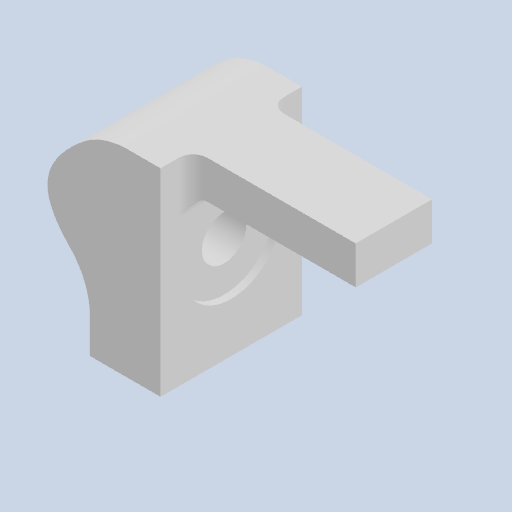
# Autodesk Inventor part: upor
Saved by Autodesk Inventor 2022 (Build 260153000, 153)
## iProperties
Created: 2024-12-11
Part Number: upor
Material: Типовые
Document SubType Name: Modeling
Designer: Andrey
Density: 1 g/cm^3
Appearance: По умолчанию
Author: Andrey
Autodesk Inventor part; units mm, degrees
ref_plane "YZ Plane" through (0, 0, 0) normal (1, 0, 0) x (0, 1, 0)
ref_plane "XZ Plane" through (0, 0, 0) normal (0, 1, 0) x (-1, 0, 0)
ref_plane "XY Plane" through (0, 0, 0) normal (0, 0, 1) x (1, 0, 0)
sketch "Эскиз1" plane through (0, 0, 0) normal (0, 0, 1) x (1, 0, 0)
  spline S0 degree 2 poles (0, -10.75) (-6, -5.75) (0, -0.75) knots -1 -1 -1 0 0 0
  circle A0 centre (31, -8.75) radius 2.1
  circle A1 centre (0.3533, 10.75) radius 2.1
  circle A2 centre (-6.5719, -8.75) radius 2.1
  arc A3 (26, -0.75) -> (0.0249, 0.0543) centre (13, -0.75) ccw
  line L0 (26, -0.75) -> (26, -14.75)
  line L1 (26, -14.75) -> (42.8533, -14.75)
  line L2 (42.8533, -14.75) -> (25.4056, 8.5426)
  arc A4 (25.4056, 8.5426) -> (13, 14.75) centre (13, -0.75) ccw
  line L3 (13, 14.75) -> (-7.8522, 14.75)
  line L4 (-7.8522, 14.75) -> (-8.8, 13.8022)
  arc A5 (-8.8, 13.8022) -> (-9.3554, 12.7353) centre (-7.3858, 12.388) ccw
  line L5 (-9.3554, 12.7353) -> (-9.4563, 12.1627)
  line L6 (-9.4563, 12.1627) -> (-3.6467, 12.1627)
  line L7 (-3.6467, 12.1627) -> (-3.6467, 9.9627)
  line L8 (-3.6467, 9.9627) -> (-9.8443, 9.9627)
  line L9 (-9.8443, 9.9627) -> (-13.8491, -12.75)
  line L10 (-13.8491, -12.75) -> (-7.0093, -12.75)
  line L11 (-7.0093, -12.75) -> (-7.0093, -14.75)
  line L12 (-7.0093, -14.75) -> (0, -14.75)
  line L13 (0, -14.75) -> (0, -11.6512)
  line L14 (1.5, -14.75) -> (26, -14.75)
  line L15 (0.9603, -9.5977) -> (1.5, -10.0794)
  line L16 (1.5, -10.0794) -> (1.5, -14.75)
  line L17 (0.9603, -1.9023) -> (2.3298, -0.75)
  line L18 (2.3298, -0.75) -> (26, -0.75)
  spline S1 degree 3 poles (0.0249, 0.0543) (0.0092, -0.1986) (-0.0544, -0.4464) (-0.2708, -0.9048) (-0.4215, -1.1114) (-0.6069, -1.2843) knots 0 0 0 0 0.5 0.5 1 1 1 1
  spline S2 degree 3 poles (-0.6318, -10.1924) (-0.4418, -10.3706) (-0.2885, -10.5841) (-0.1211, -10.951) (-0.0759, -11.0869) (-0.0153, -11.366) (0, -11.5084) (0, -11.6512) knots 0 0 0 0 0.476947 0.476947 0.738474 0.738474 1 1 1 1
  spline S3 degree 2 poles (-0.6318, -10.1924) (-5.3806, -5.7383) (-0.6069, -1.2843) knots -0.944242 -0.944242 -0.944242 -0.053426 -0.053426 -0.053426
  line L19 (1.5, -14.75) -> (6.5, -14.75)
  line L20 (6.5, -14.75) -> (6.5, -0.75)
  spline S4 degree 5 poles (0.9603, -9.5977) (0.5187, -9.2297) (0.0945, -8.8388) (-0.3025, -8.4229) (-0.9009, -7.6836) (-1.3123, -6.8331) (-1.4364, -6.4831) (-1.5637, -5.75) (-1.4364, -5.0169) (-1.3123, -4.6669) (-0.9009, -3.8164) (-0.3025, -3.0771) (0.0945, -2.6612) (0.5187, -2.2703) (0.9603, -1.9023) knots 0 0 0 0 0 0 0.305403 0.305403 0.305403 0.5 0.5 0.5 0.694597 0.694597 0.694597 1 1 1 1 1 1
  point P0 (0, 0)
  dimension "d0" = 1.5
  dimension "d2" = 1.5
  dimension "d12" = 5
  constraints: 14 end point, 3 perpendicular, 2 point on line, 1 collinear, 1 vertical alignment, 2 other
  measures "d2" distance between parallel lines of L13 L16
  measures "d12" distance of L14.start L19.end
extrude "Выдавливание1" add sketch "Эскиз1" against normal blind 10 contours L20 L14 L16 L15 S4 L17 L18
fillet "Сопряжение2" radius 5 2 edges at (1.5, -10.0794, -5) (2.3298, -0.75, -5)
fillet_without_effect "Сопряжение3"
sketch "Эскиз3" plane through (6.5, -14.75, 0) normal (1, 0, 0) x (0, 0, -1)
  line L0 (0, 0) -> (0, 14) projected
  line L1 (0, 0) -> (10, 0) projected
  line L2 (10, 14) -> (10, 0) projected
  line L3 (0, 14) -> (10, 14) projected
  line L4 (0, 14) -> (10, 14) projected
  line L5 (5, 14) -> (5, 0)
  line L6 (0, 0) -> (10, 0) projected
  circle A0 centre (5, 7) radius 1.575
  point P0 (0, 14.75)
  dimension "d13" = 3.15
  constraints: 3 midpoint, 2 end point, 1 centre point
  measures "d13" diameter of A0
extrude "Выдавливание3" cut sketch "Эскиз3" against normal blind 5 contours A0 L5 | L5 A0
chamfer "Фаска1" distance 0.7 angle 45 1 edges at (1.5, -7.75, -3.425)
sketch "Эскиз4" plane through (6.5, -14.75, 0) normal (1, 0, 0) x (0, 0, -1)
  line L0 (9, 14) -> (10, 14) projected
  line L1 (10, 0) -> (10, 14) projected
  line L2 (0, 0) -> (10, 0) projected
  line L3 (0, 14) -> (0, 0) projected
  line L4 (0, 14) -> (1, 14) projected
  circle A0 centre (5, 7) radius 2.1 projected
  line L5 (7.7, 11.3) -> (2.3, 11.3)
  line L6 (2.3, 11.3) -> (2.3, 14.3)
  line L7 (2.3, 14.3) -> (-0.3, 14.3)
  line L8 (-0.3, 14.3) -> (-0.3, -0.3)
  line L9 (-0.3, -0.3) -> (10.3, -0.3)
  line L10 (10.3, -0.3) -> (10.3, 14.3)
  line L11 (10.3, 14.3) -> (7.7, 14.3)
  line L12 (7.7, 14.3) -> (7.7, 11.3)
  line L13 (0, 14) -> (10, 14) projected
  line L14 (1, 10) -> (1, 14) projected
  line L15 (9, 10) -> (1, 10) projected
  line L16 (9, 14) -> (9, 10) projected
  point P0 (0, 14.75)
  point P1 (2, 14)
  point P2 (8, 14)
  point P3 (7.7, 14)
  point P4 (2.3, 14)
  constraints: 16 end point, 4 other
extrude "Выдавливание4" add sketch "Эскиз4" along normal blind 11.5 contours L12 L5 L6 L13
fillet "Сопряжение4" radius 1 3 edges at (6.5, -2.1, -7.7) (6.5, -3.45, -5) (6.5, -2.1, -2.3)
sketch "Эскиз5" plane through (6.5, -14.75, 0) normal (1, 0, 0) x (0, 0, -1)
  circle A0 centre (5, 7) radius 1.575 projected
  line L0 (8.7, 10.3) -> (8.7, 14) projected
  line L1 (1.3, 10.3) -> (8.7, 10.3) projected
  line L2 (1.3, 14) -> (1.3, 10.3) projected
  line L3 (0, 14) -> (1.3, 14) projected
  line L4 (0, 0) -> (0, 14) projected
  line L5 (0, 0) -> (10, 0) projected
  line L6 (10, 14) -> (10, 0) projected
  line L7 (8.7, 14) -> (10, 14) projected
  circle A1 centre (5, 7) radius 1.575 projected
  circle A2 centre (5, 7) radius 3.5
  point P0 (0, 14.75)
  point P1 (3.8338, 10.3)
  point P2 (6.1662, 10.3)
  dimension "d23" = 7
  constraints: 1 centre point, 1 coincident
  measures "d23" diameter of A2
extrude "Выдавливание5" cut sketch "Эскиз5" along normal mid plane 1 contours A0 | A2 L1 | L1 A2
